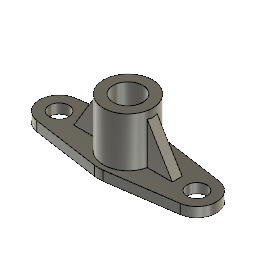
Semana3_Desafio3 v1 (Autodesk Fusion 360 design; units mm, degrees)
Autodesk Fusion 360 part; units mm, degrees
sketch "Sketch1" plane through (0, 0, 0) normal (0, 0, 1) x (1, 0, 0)
  circle A0 centre (0, 0) radius 12.5
  circle A1 centre (0, 0) radius 7.5
  circle A2 centre (-35, 0) radius 5
  circle A3 centre (35, 0) radius 5
  line L0 (-60, 0) -> (60, 0) construction
  line L1 (-35, 0) -> (-35, 14) construction
  line L2 (-35, 14) -> (-35, -13) construction
  line L3 (35, 0) -> (35, 14) construction
  line L4 (35, 14) -> (35, -13) construction
  line L5 (-36.4286, -9.8974) -> (-2.1429, -14.8461)
  line L6 (36.4286, -9.8974) -> (2.1429, -14.8461)
  line L7 (36.4286, 9.8974) -> (2.1429, 14.8461)
  line L8 (-36.4286, 9.8974) -> (-2.1429, 14.8461)
  arc A4 (-35, 10) -> (-35, -10) centre (-35, 0) ccw
  arc A5 (35, -10) -> (35, 10) centre (35, 0) ccw
  arc A6 (-2.1429, -14.8461) -> (2.1429, -14.8461) centre (0, 0) ccw
  arc A7 (2.1429, 14.8461) -> (-2.1429, 14.8461) centre (0, 0) ccw
  dimension "d1" = 30
  dimension "d2" = 25
  dimension "d3" = 15
  dimension "d4" = 10
  dimension "d5" = 10
  dimension "d6" = 20
  dimension "d7" = 20
  dimension "d8" = 35
  dimension "d9" = 35
  constraint coincident A0.centre A1.centre
  constraint concentric A0 A1
  constraint concentric A2 A4
  constraint concentric A3 A5
  constraint collinear A0.centre A2.centre A3.centre
  constraint horizontal L0
  constraint coincident A2.centre L1.start
  constraint perpendicular L0 L1
  constraint perpendicular L0 L2
  constraint coincident A3.centre L3.start
  constraint perpendicular L0 L3
  constraint parallel L3 L4
  constraint tangent L8 A4
  constraint tangent L8 A6
  constraint tangent L7 A6
  constraint tangent L7 A5
  constraint tangent L5 A4
  constraint tangent L5 A6
  constraint tangent L6 A6
  constraint tangent L6 A5
  constraint coincident L7.end A6
  constraint coincident L7.start A5
  constraint coincident L6.start A5
  constraint coincident L8.start A4
  constraint coincident L5.start A4
  constraint coincident L1 A4.start
  constraint coincident L2 A4.end
  constraint coincident L3 A5.end
  constraint coincident L4 A5.start
  constraint concentric A6 A7
  measures "d1" diameter of A6
  measures "d2" diameter of A0
  measures "d3" diameter of A1
  measures "d4" diameter of A2
  measures "d5" diameter of A3
  measures "d6" diameter of A4
  measures "d7" diameter of A5
  measures "d8" distance of A0.centre A2.centre
  measures "d9" distance of A0.centre A3.centre
extrude "Extrude1" add sketch "Sketch1" along normal blind 5 contours L5 L6 L7 L8 A4 A5 A6 A7
sketch "Sketch2" plane through (0, 0, 0) normal (0, 0, 1) x (1, 0, 0)
  circle A0 centre (0, 0) radius 12.5
  circle A1 centre (0, 0) radius 7.5
  dimension "d12" = 25
  dimension "d13" = 15
  constraint coincident A0.centre A1.centre
  measures "d12" diameter of A0
  measures "d13" diameter of A1
extrude "Extrude2" add sketch "Sketch2" along normal blind 30
sketch "Sketch6" plane through (0, 0, 0) normal (0, 1, 0) x (1, 0, 0)
  line L0 (-10, -5) -> (-25, -5)
  line L1 (-25, -5) -> (-10, -30)
  line L2 (-10, -30) -> (-10, -5)
  line L3 (10, -5) -> (25, -5)
  line L4 (25, -5) -> (10, -30)
  line L5 (10, -30) -> (10, -5)
  line L6 (-36.4286, -5) -> (-2.1429, -5)
  line L7 (2.1429, -5) -> (36.4286, -5)
  dimension "d27" = 10
  dimension "d28" = 10
  dimension "d29" = 15
  dimension "d30" = 15
  dimension "d31" = 25
  constraint horizontal L0
  constraint perpendicular L0 L2
  constraint perpendicular L2 L3
  constraint perpendicular L3 L5
  constraint equal L2 L5
  constraint collinear L0 L6
  constraint collinear L3 L7
  measures "d27" horizontal distance of origin L0.start
  measures "d28" horizontal distance of origin L3.start
  measures "d29" distance of L0.start L0.end
  measures "d30" distance of L3.start L3.end
  measures "d31" distance of L0.start L1.end
extrude "Extrude4" add sketch "Sketch6" along normal blind 2.5 and the other way blind 2.5
